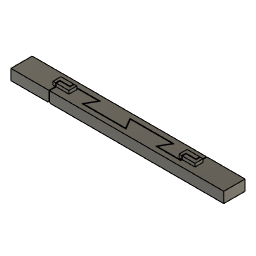
Straight-Track-Parametric (Autodesk Fusion 360 archive; units mm, degrees)
design "Track Joint Parametric"
Autodesk Fusion 360 part; units mm, degrees
sketch "Sketch1" plane through (0, 0, 0) normal (0, 0, 1) x (1, 0, 0)
  line L0 (20, -2) -> (-20, -2)
  line L1 (-20, -2) -> (-20, 2)
  line L2 (-20, 2) -> (20, 2)
  line L3 (20, 2) -> (20, -2)
  line L4 (20, -2) -> (-20, 2) construction
  line L5 (-20, -2) -> (20, 2) construction
  line L6 (0, 0) -> (0, -2) construction
  line L7 (0, 0) -> (0, 2) construction
  line L8 (-12.45, 2) -> (-12.45, -2) construction
  line L9 (-11.25, 2) -> (-11.25, -2) construction
  line L10 (-12.75, 2) -> (-12.75, -2)
  line L11 (-10.95, 2) -> (-10.95, -2)
  line L12 (-10.85, 2) -> (-10.85, -2)
  line L13 (-12.85, 2) -> (-12.85, -2)
  line L14 (-11.85, 2) -> (-11.85, -2) construction
  line L15 (-20, 0.05) -> (20, 0.05)
  line L16 (20, -0.05) -> (-20, -0.05)
  line L17 (-20, 0) -> (20, 0) construction
  line L18 (0.5774, -1) -> (-0.5774, 1) construction
  line L19 (0.5774, -1) -> (-7.5, -1) construction
  line L20 (-7.5, -1) -> (-6.3453, 1) construction
  line L21 (-6.3453, 1) -> (-10.95, 1) construction
  line L22 (-0.5774, 1) -> (7.5, 1) construction
  line L23 (7.5, 1) -> (6.3453, -1) construction
  line L24 (6.3453, -1) -> (10.95, -1) construction
  line L25 (-3.4613, -1) -> (-3.4613, 1.05) construction
  line L26 (3.4613, 1) -> (3.4613, -1.05) construction
  line L27 (-6.2587, 1.05) -> (-10.95, 1.05)
  line L28 (-7.4134, -0.95) -> (-6.2587, 1.05)
  line L29 (0.4907, -0.95) -> (-7.4134, -0.95)
  line L30 (0.4907, -0.95) -> (-0.664, 1.05)
  line L31 (-0.664, 1.05) -> (7.5866, 1.05)
  line L32 (7.5866, 1.05) -> (6.4319, -0.95)
  line L33 (6.4319, -0.95) -> (10.95, -0.95)
  line L34 (12.85, 2) -> (12.85, -2)
  line L35 (12.75, 2) -> (12.75, -2)
  line L36 (12.45, 2) -> (12.45, -2) construction
  line L37 (11.25, 2) -> (11.25, -2) construction
  line L38 (10.95, 2) -> (10.95, -2)
  line L39 (10.85, 2) -> (10.85, -2)
  line L40 (-6.4319, 0.95) -> (-10.95, 0.95)
  line L41 (-7.5866, -1.05) -> (-6.4319, 0.95)
  line L42 (0.664, -1.05) -> (-7.5866, -1.05)
  line L43 (0.664, -1.05) -> (-0.4907, 0.95)
  line L44 (-0.4907, 0.95) -> (7.4134, 0.95)
  line L45 (7.4134, 0.95) -> (6.2587, -1.05)
  line L46 (6.2587, -1.05) -> (10.95, -1.05)
  line L47 (11.85, 2) -> (11.85, -2) construction
  line L48 (-10.35, -0.75) -> (-13.35, -0.75)
  line L49 (-13.35, -0.75) -> (-13.35, 0.75)
  line L50 (-13.35, 0.75) -> (-10.35, 0.75)
  line L51 (-10.35, 0.75) -> (-10.35, -0.75)
  line L52 (-10.35, -0.75) -> (-13.35, 0.75) construction
  line L53 (-13.35, -0.75) -> (-10.35, 0.75) construction
  line L54 (13.35, -0.75) -> (10.35, -0.75)
  line L55 (10.35, -0.75) -> (10.35, 0.75)
  line L56 (10.35, 0.75) -> (13.35, 0.75)
  line L57 (13.35, 0.75) -> (13.35, -0.75)
  line L58 (13.35, -0.75) -> (10.35, 0.75) construction
  line L59 (10.35, -0.75) -> (13.35, 0.75) construction
  point P0 (-11.85, 0)
  point P1 (11.85, 0)
  dimension "d1" = 4
  dimension "d2" = 40
  dimension "d16" = 0.1
  dimension "d57" = 0.1
  dimension "d60" = 2
  dimension "d61" = 30
  dimension "d62" = 15
  dimension "d63" = 0.05
  dimension "d69" = 1.2
  dimension "d70" = 1.8
  dimension "d73" = 22.5
  dimension "d74" = -0.05
  dimension "d113" = 3
  dimension "d114" = 1.5
  constraint horizontal L0
  constraint perpendicular L0 L1
  constraint parallel L0 L2
  constraint parallel L1 L3
  constraint coincident L4 L6.start
  constraint coincident L5 L6.start
  constraint coincident L6.start L7.start
  constraint midpoint L0 L6.end
  constraint midpoint L2 L7.end
  constraint coincident L0 L8.end
  constraint perpendicular L0 L8
  constraint coincident L2 L9.start
  constraint coincident L0 L9.end
  constraint perpendicular L0 L9
  constraint coincident L2 L10.start
  constraint coincident L2 L11.start
  constraint perpendicular L0 L10
  constraint perpendicular L0 L11
  constraint coincident L2 L12.start
  constraint coincident L2 L13.start
  constraint coincident L2 L14.start
  constraint coincident L0 L14.end
  constraint symmetric L8 L9 L14
  constraint coincident L1 L15.start
  constraint coincident L3 L15.end
  constraint perpendicular L3 L15
  constraint coincident L3 L16.start
  constraint coincident L1 L16.end
  constraint perpendicular L1 L16
  constraint midpoint L1 L17.start
  constraint midpoint L3 L17.end
  constraint symmetric L15 L16 L17
  constraint coincident L0 L13.end
  constraint coincident L0 L10.end
  constraint coincident L0 L11.end
  constraint coincident L0 L12.end
  constraint midpoint L6.start L18
  constraint horizontal L21
  constraint horizontal L19
  constraint horizontal L22
  constraint horizontal L24
  constraint collinear L19 L24
  constraint collinear L21 L22
  constraint equal L19 L22
  constraint midpoint L19 L25.start
  constraint perpendicular L19 L25
  constraint midpoint L22 L26.start
  constraint perpendicular L22 L26
  constraint symmetric L18 L20 L25
  constraint symmetric L18 L23 L26
  constraint coincident L2 L8.start
  constraint symmetric L10 L11 L14
  constraint symmetric L6 L8.start L36.start
  constraint symmetric L6 L8.end L36.end
  constraint symmetric L6 L9.start L37.start
  constraint symmetric L6 L9.end L37.end
  constraint symmetric L6 L10.start L35.start
  constraint symmetric L6 L10.end L35.end
  constraint symmetric L6 L11.start L38.start
  constraint symmetric L6 L11.end L38.end
  constraint symmetric L6 L12.start L39.start
  constraint symmetric L6 L12.end L39.end
  constraint symmetric L6 L13.start L34.start
  constraint symmetric L6 L13.end L34.end
  constraint horizontal L25.end L30.end
  constraint horizontal L26.end L42.start
  constraint coincident L24.end L38
  constraint coincident L11 L21.end
  constraint coincident L2 L47.start
  constraint coincident L0 L47.end
  constraint perpendicular L0 L47
  constraint symmetric L36 L37 L47
  constraint horizontal L48
  constraint perpendicular L48 L49
  constraint parallel L48 L50
  constraint parallel L49 L51
  constraint coincident L52 P0
  constraint coincident L53 P0
  constraint midpoint L14 P0
  constraint horizontal L54
  constraint perpendicular L54 L55
  constraint parallel L54 L56
  constraint parallel L55 L57
  constraint coincident L58 P1
  constraint coincident L59 P1
  constraint midpoint L47 P1
  constraint equal L49 L55
  constraint equal L48 L54
  measures "d1" distance of L0.start L2.end
  measures "d2" distance of L1.end L2.end
  measures "d16" distance of L11 L12
  measures "d57" distance of L15 L16
  measures "d60" vertical distance of L18.start L18.end
  measures "d61" angle of L6 L18
  measures "d62" horizontal distance of L19.end L22.end
  measures "d69" distance of L8 L9
  measures "d70" distance of L10 L11
  measures "d73" distance of L9 L37
  measures "d113" distance of L48.start L48.end
  measures "d114" distance of L48.end L49.end
sketch "Sketch2" plane through (0, 0, 0) normal (0, 1, 0) x (1, 0, 0)
  line L0 (12.75, -0.3) -> (12.75, 0)
  line L1 (12.75, 0) -> (10.95, 0)
  line L2 (10.95, 0) -> (10.95, -0.3)
  line L3 (11.25, -2.4) -> (12.45, -2.4)
  line L4 (12.45, -2.4) -> (12.45, -1.8)
  line L5 (11.25, -1.8) -> (11.25, -2.4)
  line L6 (11.25, -1.8) -> (11.45, -1.8)
  line L7 (11.45, -1.8) -> (11.45, -0.3)
  line L8 (11.45, -0.3) -> (10.95, -0.3)
  line L9 (12.75, -0.3) -> (12.25, -0.3)
  line L10 (12.25, -0.3) -> (12.25, -1.8)
  line L11 (12.25, -1.8) -> (12.45, -1.8)
  line L12 (11.85, 0) -> (11.85, -2.4) construction
  line L13 (-12.45, -1.8) -> (-12.45, -2.4)
  line L14 (-11.85, 0) -> (-11.85, -2.4) construction
  line L15 (-10.95, 0) -> (-12.75, 0)
  line L16 (-12.45, -2.4) -> (-11.25, -2.4)
  line L17 (-11.45, -1.8) -> (-11.25, -1.8)
  line L18 (-12.75, 0) -> (-12.75, -0.3)
  line L19 (-11.25, -2.4) -> (-11.25, -1.8)
  line L20 (-10.95, -0.3) -> (-11.45, -0.3)
  line L21 (-11.45, -0.3) -> (-11.45, -1.8)
  line L22 (-12.25, -0.3) -> (-12.75, -0.3)
  line L23 (-10.95, -0.3) -> (-10.95, 0)
  line L24 (-12.45, -1.8) -> (-12.25, -1.8)
  line L25 (-12.25, -1.8) -> (-12.25, -0.3)
  point P0 (-11.85, 0)
  point P1 (11.85, 0)
  point P2 (12.45, 0)
  point P3 (12.75, 0)
  point P4 (-11.25, 0)
  point P5 (-10.95, 0)
  dimension "d77" = 0.3
  dimension "d85" = 1.2
  dimension "d87" = 0.6
  dimension "d88" = 0.8
  dimension "d94" = 2.4
  constraint vertical L0
  constraint horizontal L1
  constraint vertical L2
  constraint midpoint L1 P1
  constraint coincident L0.end L1.start
  constraint horizontal L3
  constraint vertical L4
  constraint vertical L5
  constraint coincident P2 L4
  constraint perpendicular L5 L6
  constraint perpendicular L6 L7
  constraint perpendicular L7 L8
  constraint perpendicular L0 L9
  constraint perpendicular L9 L10
  constraint coincident P1 L12.start
  constraint midpoint L3 L12.end
  constraint perpendicular L3 L12
  constraint symmetric L7 L10 L12
  constraint perpendicular L10 L11
  constraint collinear L8 L9
  constraint vertical L23
  constraint horizontal L15
  constraint vertical L18
  constraint coincident P5 L15.start
  constraint horizontal L16
  constraint vertical L19
  constraint vertical L13
  constraint coincident P4 L19
  constraint perpendicular L13 L24
  constraint perpendicular L24 L25
  constraint perpendicular L22 L25
  constraint perpendicular L20 L23
  constraint perpendicular L20 L21
  constraint midpoint L14.end L16
  constraint perpendicular L14 L16
  constraint perpendicular L17 L21
  constraint collinear L20 L22
  constraint midpoint P0 L15
  constraint collinear L6 L11
  constraint equal L10 L21
  constraint equal L3 L16
  constraint coincident P0 L14.start
  constraint equal L11 L17
  constraint equal L9 L20
  constraint equal L0 L23
  constraint equal L4 L19
  measures "d77" distance of L0.start L0.end
  measures "d85" distance of L3.start L3.end
  measures "d87" distance of L3.end L4.end
  measures "d88" distance of L7 L10
  measures "d94" distance of L1 L3
extrude "Extrude2" add sketch "Sketch1" against normal blind 2 contours L15 L35 L38 L56 | L16 L39 L54 L55 | L16 L32 L33 L39 L54 L55 | L2 L35 L38 L56 | L15 L16 L39 L55 | L15 L38 L39 L56 | L2 L38 L39 L56 | L15 L16 L32 L55 | L15 L39 L55 L56 | L2 L12 L15 L27 L28 L30 L31 L32 L39 L55 L56 | L0 L1 L13 L16 L48 L49 | L2 L11 L12 L27 | L13 L16 L48 L49 | L10 L11 L15 L50 | L16 L28 L29 L30 | L15 L16 L28 L30 | L2 L10 L11 L50 | L1 L15 L16 L49 | L13 L15 L16 L49 | L10 L13 L15 L50 | L2 L10 L13 L50 | L1 L2 L13 L15 L49 L50 | L13 L15 L49 L50 makes body 1
extrude "Extrude3" add sketch "Sketch1" along normal blind 0.6 contours L15 L35 L38 L56 | L16 L39 L54 L55 | L15 L16 L39 L55 | L15 L38 L39 L56 | L15 L39 L55 L56 | L13 L16 L48 L49 | L10 L11 L15 L50 | L13 L15 L16 L49 | L10 L13 L15 L50 | L13 L15 L49 L50 bodies 1
extrude "Extrude1" add sketch "Sketch1" against normal up to surface (2 mm away) separate body contours L0 L3 L16 L34 L54 L57 | L0 L34 L35 L54 | L3 L15 L16 L57 | L0 L35 L38 L54 | L16 L34 L35 L54 | L16 L34 L54 L57 | L2 L3 L15 L34 L56 L57 | L15 L16 L34 L57 | L0 L38 L39 L46 | L16 L35 L38 L54 | L15 L34 L56 L57 | L0 L12 L16 L39 L41 L42 L43 L45 L46 L48 L51 | L0 L11 L12 L48 | L0 L10 L11 L48 | L11 L12 L16 L48 | L12 L16 L48 L51 | L10 L11 L16 L48 | L12 L15 L16 L51 | L15 L16 L43 L45 | L12 L15 L50 L51 | L15 L16 L41 L51 | L15 L43 L44 L45 | L12 L15 L40 L41 L50 L51 makes body 2 in component "Join 2"
extrude "Extrude2'" add sketch "Sketch1" along normal up to surface (0.6 mm away) contours L16 L34 L35 L54 | L16 L34 L54 L57 | L15 L16 L34 L57 | L16 L35 L38 L54 | L15 L34 L56 L57 | L11 L12 L16 L48 | L12 L16 L48 L51 | L10 L11 L16 L48 | L12 L15 L16 L51 | L12 L15 L50 L51 bodies 2 in component "Join 2"
chamfer "Chamfer2" distance 0.2 angle 45 13 edges at (-11.9, 0.05, -2) (-12.85, -0.975, -2) (-10.95, 0.55, -2) (-8.6043, 1.05, -2) (-6.836, 0.05, -2) (-3.4613, -0.95, -2) (-0.0866, 0.05, -2) (3.4613, 1.05, -2) (7.0093, 0.05, -2) (8.641, -0.95, -2) (10.85, -0.45, -2) (11.8, 0.05, -2) (12.75, 1.025, -2) on bodies 1
chamfer "Chamfer1" distance 0.2 angle 45 13 edges at (-8.641, 0.95, -2) (-10.85, 0.45, -2) (-11.8, -0.05, -2) (-12.75, -1.025, -2) (-7.0093, -0.05, -2) (-3.4613, -1.05, -2) (0.0866, -0.05, -2) (3.4613, 0.95, -2) (6.836, -0.05, -2) (8.6043, -1.05, -2) (10.95, -0.55, -2) (11.9, -0.05, -2) (12.85, 0.975, -2) on bodies 2 in component "Join 2"
component "Join 2" placed x (1, 0, 0) y (0, 1, 0) z (0, 0, 1) at (0, 0, 0)
equation "d1 = d62 / 3.75"
equation "d2 = d1 * 10"
equation "d57 = Tollerance"
equation "d60 = d1 / 2"
equation "d62 = d73 / 1.5"
equation "d69 = d73 / 18.75"
equation "d70 = d69 * 1.5"
equation "d73 = Gauge"
equation "d77 = d85 / 4"
equation "d87 = d85 / 2"
equation "d88 = d85 / 3 * 2"
equation "d94 = d85 * 2"
equation "Gauge = 22.5 mm"
equation "SleeperThickness = 2 mm"
equation "Tollerance = 0.1 mm"
equation "d105 = -SleeperThickness"
equation "SleeperSpcing = Gauge / 1.5"
equation "d113 = d69 * 2.5"
equation "d114 = d113 / 2"
equation "d115 = Gauge / 37.5"
named bodies: "Joint 1"
